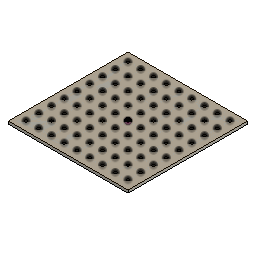
dogs (Autodesk Fusion 360 archive; units mm, degrees)
design "Board"
Autodesk Fusion 360 part; units mm, degrees
sketch "Skizze2" plane through (0, 0, 0) normal (0, 0, 1) x (1, 0, 0) in component "Board"
  line L0 (450, 450) -> (-450, 450)
  line L1 (-450, 450) -> (-450, -450)
  line L2 (-450, -450) -> (450, -450)
  line L3 (450, -450) -> (450, 450)
  line L4 (450, 450) -> (-450, -450) construction
  line L5 (-450, 450) -> (450, -450) construction
  dimension "d4" = 900
  dimension "d5" = 900
  constraint perpendicular L0 L1
  constraint parallel L0 L2
  constraint parallel L1 L3
  constraint horizontal L0
  constraint coincident L4 origin
  constraint coincident L5 origin
  measures "d4" distance of L1.end L2.end
  measures "d5" distance of L0.end L1.end
extrude "Extrusion1" add sketch "Skizze2" along normal blind 21 makes body 1 in component "Board"
sketch "Skizze3" plane through (0, 0, 21) normal (0, 0, 1) x (-1, 0, 0) in component "Board"
  line L0 (-450, 450) -> (-450, -450)
  line L1 (-450, -450) -> (450, -450)
  line L2 (450, -450) -> (450, 450)
  line L3 (450, 450) -> (-450, 450)
  circle A0 centre (384, -384) radius 10
  circle A1 centre (288, -384) radius 10
  circle A2 centre (192, -384) radius 10
  circle A3 centre (96, -384) radius 10
  circle A4 centre (0, -384) radius 10
  circle A5 centre (-96, -384) radius 10
  circle A6 centre (-192, -384) radius 10
  circle A7 centre (-288, -384) radius 10
  circle A8 centre (-384, -384) radius 10
  circle A9 centre (384, -288) radius 10
  circle A10 centre (288, -288) radius 10
  circle A11 centre (192, -288) radius 10
  circle A12 centre (96, -288) radius 10
  circle A13 centre (0, -288) radius 10
  circle A14 centre (-96, -288) radius 10
  circle A15 centre (-192, -288) radius 10
  circle A16 centre (-288, -288) radius 10
  circle A17 centre (-384, -288) radius 10
  circle A18 centre (384, -192) radius 10
  circle A19 centre (288, -192) radius 10
  circle A20 centre (192, -192) radius 10
  circle A21 centre (96, -192) radius 10
  circle A22 centre (0, -192) radius 10
  circle A23 centre (-96, -192) radius 10
  circle A24 centre (-192, -192) radius 10
  circle A25 centre (-288, -192) radius 10
  circle A26 centre (-384, -192) radius 10
  circle A27 centre (384, -96) radius 10
  circle A28 centre (288, -96) radius 10
  circle A29 centre (192, -96) radius 10
  circle A30 centre (96, -96) radius 10
  circle A31 centre (0, -96) radius 10
  circle A32 centre (-96, -96) radius 10
  circle A33 centre (-192, -96) radius 10
  circle A34 centre (-288, -96) radius 10
  circle A35 centre (-384, -96) radius 10
  circle A36 centre (384, 0) radius 10
  circle A37 centre (288, 0) radius 10
  circle A38 centre (192, 0) radius 10
  circle A39 centre (96, 0) radius 10
  circle A40 centre (0, 0) radius 10
  circle A41 centre (-96, 0) radius 10
  circle A42 centre (-192, 0) radius 10
  circle A43 centre (-288, 0) radius 10
  circle A44 centre (-384, 0) radius 10
  circle A45 centre (384, 96) radius 10
  circle A46 centre (288, 96) radius 10
  circle A47 centre (192, 96) radius 10
  circle A48 centre (96, 96) radius 10
  circle A49 centre (0, 96) radius 10
  circle A50 centre (-96, 96) radius 10
  circle A51 centre (-192, 96) radius 10
  circle A52 centre (-288, 96) radius 10
  circle A53 centre (-384, 96) radius 10
  circle A54 centre (384, 192) radius 10
  circle A55 centre (288, 192) radius 10
  circle A56 centre (192, 192) radius 10
  circle A57 centre (96, 192) radius 10
  circle A58 centre (0, 192) radius 10
  circle A59 centre (-96, 192) radius 10
  circle A60 centre (-192, 192) radius 10
  circle A61 centre (-288, 192) radius 10
  circle A62 centre (-384, 192) radius 10
  circle A63 centre (384, 288) radius 10
  circle A64 centre (288, 288) radius 10
  circle A65 centre (192, 288) radius 10
  circle A66 centre (96, 288) radius 10
  circle A67 centre (0, 288) radius 10
  circle A68 centre (-96, 288) radius 10
  circle A69 centre (-192, 288) radius 10
  circle A70 centre (-288, 288) radius 10
  circle A71 centre (-384, 288) radius 10
  circle A72 centre (384, 384) radius 10
  circle A73 centre (288, 384) radius 10
  circle A74 centre (192, 384) radius 10
  circle A75 centre (96, 384) radius 10
  circle A76 centre (0, 384) radius 10
  circle A77 centre (-96, 384) radius 10
  circle A78 centre (-192, 384) radius 10
  circle A79 centre (-288, 384) radius 10
  circle A80 centre (-384, 384) radius 10
  dimension "d10" = 20
  dimension "d15" = -96
  dimension "d16" = 96
  dimension "d40" = 66
  dimension "d41" = 66
  constraint coincident A40.centre origin
  measures "d10" diameter of A0
  measures "d40" distance of L1 A8.centre
  measures "d41" distance of L0 A8.centre
sketch "Skizze1" plane through (0, 0, 0) normal (0, 0, -1) x (-1, 0, 0) in component "Legs"
  line L0 (-228, 228) -> (-348, 228)
  line L1 (-348, 228) -> (-348, 348)
  line L2 (-348, 348) -> (-228, 348)
  line L3 (-228, 348) -> (-228, 228)
  line L4 (-228, 228) -> (-348, 348) construction
  line L5 (-348, 228) -> (-228, 348) construction
  line L6 (-233, 233) -> (-343, 233)
  line L7 (-343, 233) -> (-343, 343)
  line L8 (-343, 343) -> (-233, 343)
  line L9 (-233, 343) -> (-233, 233)
  line L10 (228, 348) -> (348, 348)
  line L11 (233, 343) -> (343, 343)
  line L12 (348, 348) -> (348, 228)
  line L13 (343, 343) -> (343, 233)
  line L14 (343, 233) -> (233, 233)
  line L15 (348, 228) -> (228, 228)
  line L16 (228, 228) -> (228, 348)
  line L17 (233, 233) -> (233, 343)
  line L18 (-348, -228) -> (-228, -228)
  line L19 (-343, -233) -> (-233, -233)
  line L20 (-228, -228) -> (-228, -348)
  line L21 (-233, -233) -> (-233, -343)
  line L22 (-233, -343) -> (-343, -343)
  line L23 (-228, -348) -> (-348, -348)
  line L24 (-348, -348) -> (-348, -228)
  line L25 (-343, -343) -> (-343, -233)
  line L26 (228, -228) -> (348, -228)
  line L27 (233, -233) -> (343, -233)
  line L28 (348, -228) -> (348, -348)
  line L29 (343, -233) -> (343, -343)
  line L30 (343, -343) -> (233, -343)
  line L31 (348, -348) -> (228, -348)
  line L32 (228, -348) -> (228, -228)
  line L33 (233, -343) -> (233, -233)
  line L34 (-450, 450) -> (-450, -450)
  line L35 (-450, -450) -> (450, -450)
  line L36 (450, -450) -> (450, 450)
  line L37 (450, 450) -> (-450, 450)
  point P0 (-288, 288)
  point P1 (-288, 288)
  dimension "d23" = 120
  dimension "d24" = 120
  dimension "d27" = 5
  dimension "d30" = 576
  dimension "d31" = -576
  constraint perpendicular L0 L1
  constraint parallel L0 L2
  constraint parallel L1 L3
  constraint horizontal L0
  constraint coincident L4 P1
  constraint coincident L5 P1
  constraint coincident P1 P0
  measures "d23" distance of L1.end L2.end
  measures "d24" distance of L0.end L1.end
extrude "Extrusion1'" add sketch "Skizze1" along normal blind 70 separate body contours L0 L1 L2 L3 | L6 L7 L8 L9 | L10 L12 L15 L16 | L11 L13 L14 L17 | L18 L20 L23 L24 | L19 L21 L22 L25 | L26 L28 L31 L32 | L27 L29 L30 L33 makes body 2 at (308, -268, 0) makes body 3 at (-268, 308, 0) makes body 4 at (-268, -268, 0) makes body 5 at (268, 268, 0) in component "Legs"
sketch "Skizze2 (2)" plane through (0, 0, -70) normal (0, 0, -1) x (1, 0, 0) in component "Legs"
  line L0 (-228, 348) -> (-348, 348)
  line L1 (-348, 348) -> (-348, 228)
  line L2 (-348, 228) -> (-228, 228)
  line L3 (-228, 228) -> (-228, 348)
  line L4 (-343, 343) -> (-233, 343)
  line L5 (-233, 343) -> (-233, 233)
  line L6 (-233, 233) -> (-343, 233)
  line L7 (-343, 233) -> (-343, 343)
  line L8 (233, 343) -> (343, 343)
  line L9 (233, 233) -> (233, 343)
  line L10 (343, 343) -> (343, 233)
  line L11 (343, 233) -> (233, 233)
  line L12 (-343, -233) -> (-233, -233)
  line L13 (-343, -343) -> (-343, -233)
  line L14 (-233, -233) -> (-233, -343)
  line L15 (-233, -343) -> (-343, -343)
  line L16 (233, -233) -> (343, -233)
  line L17 (233, -343) -> (233, -233)
  line L18 (343, -233) -> (343, -343)
  line L19 (343, -343) -> (233, -343)
extrude "Extrusion2" cut sketch "Skizze2 (2)" against normal blind 2 contours L4 L5 L6 L7 | L8 L9 L10 L11 | L12 L13 L14 L15 | L16 L17 L18 L19 bodies 2 3 4 5 in component "Legs"
extrude "Extrusion3" add sketch "Skizze3" against normal up to surface (21 mm away) contours A10 | A16 | A64 | A70 bodies 2 3 4 5 in component "Legs"
extrude "Extrusion3'" cut sketch "Skizze3" against normal up to surface (21 mm away) contours A10 | A16 | A64 | A70 bodies 1 in component "Board"
component "Board" placed x (1, 0, 0) y (0, 1, 0) z (0, 0, 1) at (0, 0, 0)
component "Legs" placed x (1, 0, 0) y (0, 1, 0) z (0, 0, 1) at (0, 0, 0)
equation "board_width = 900 mm"
equation "board_length = 900 mm"
equation "board_thickness = 21 mm"
equation "d4 = board_width"
equation "d5 = board_length"
equation "d6 = board_thickness"
equation "hole_dia = 20 mm"
equation "tolerance = 0.1 mm"
equation "d10 = hole_dia"
equation "leg_width = 120 mm"
equation "leg_length = 120 mm"
equation "leg_height = 70 mm"
equation "stopper_thickness = 2 mm"
equation "stopper_width = leg_width - ( stopper_offfset * 2 )"
equation "stopper_legth = leg_length - ( stopper_offfset * 2 )"
equation "d23 = leg_width"
equation "d24 = leg_length"
equation "hole_distance = 96 mm"
equation "stopper_offfset = 5 mm"
equation "d27 = stopper_offfset"
equation "d30 = hole_distance * 6"
equation "d31 = -( hole_distance * 6 )"
equation "d32 = leg_height"
equation "d34 = -stopper_thickness"
named bodies: "leg 1", "leg 3", "leg 2", "leg 4"
